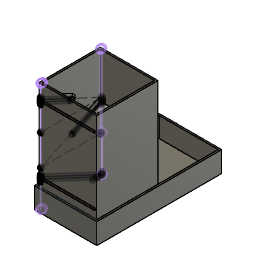
DiceTowerSlides (Autodesk Fusion 360 design; units mm, degrees)
Autodesk Fusion 360 part; units mm, degrees
sketch "Sketch1" plane through (0, 0, 0) normal (0, 1, 0) x (1, 0, 0)
  line L0 (30, 60) -> (-30, 60)
  line L1 (-30, 60) -> (-30, -60)
  line L2 (-30, -60) -> (30, -60)
  line L3 (30, -60) -> (30, 60)
  line L4 (30, 60) -> (-30, -60) construction
  line L5 (-30, 60) -> (30, -60) construction
  line L6 (28.33, 58.33) -> (-28.33, 58.33)
  line L7 (-28.33, 58.33) -> (-28.33, -58.33)
  line L8 (-28.33, -58.33) -> (28.33, -58.33)
  line L9 (28.33, -58.33) -> (28.33, 58.33)
  line L10 (28.33, 58.33) -> (-28.33, -58.33) construction
  line L11 (-28.33, 58.33) -> (28.33, -58.33) construction
  dimension "d3" = 120
  dimension "d4" = 60
  dimension "d5" = 1.67
  dimension "d6" = 1.67
  constraint horizontal L0
  constraint perpendicular L0 L1
  constraint parallel L0 L2
  constraint parallel L1 L3
  constraint coincident L4 origin
  constraint coincident L5 origin
  constraint horizontal L6
  constraint perpendicular L6 L7
  constraint parallel L6 L8
  constraint parallel L7 L9
  constraint coincident L10 origin
  constraint coincident L11 origin
  measures "d3" distance of L0.end L1.end
  measures "d4" distance of L1 L3
  measures "d5" distance of L1 L7
  measures "d6" distance of L0 L6
extrude "Extrude1" add sketch "Sketch1" along normal blind 20 makes body 1
extrude "Extrude2" add sketch "Sketch1" along normal blind 0.8 contours L6 L7 L8 L9 bodies 1
sketch "Sketch2" plane through (0, 0, 58.33) normal (0, 0, -1) x (-1, 0, 0)
  line L0 (-28.33, 0.8) -> (28.33, 0.8)
  line L1 (28.33, 0.8) -> (28.33, 20)
  line L2 (28.33, 20) -> (-28.33, 20)
  line L3 (-28.33, 20) -> (-28.33, 0.8)
sketch "Sketch2 (2)" plane through (0, 0.8, 0) normal (0, 1, 0) x (-1, 0, 0) in component "Tower"
  line L0 (-28.33, 58.33) -> (-28.33, -58.33)
  line L1 (-28.33, -58.33) -> (28.33, -58.33)
  line L2 (28.33, -58.33) -> (28.33, 58.33)
  line L3 (28.33, 58.33) -> (-28.33, 58.33)
  line L4 (28.33, 58.33) -> (-28.33, 58.33)
  line L5 (-28.33, 58.33) -> (28.33, 58.33) construction
  line L6 (28.33, 58.33) -> (28.33, -1.67) construction
  line L7 (28.33, -1.67) -> (-28.33, -1.67) construction
  line L8 (-28.33, -1.67) -> (-28.33, 58.33) construction
  line L9 (27.73, 57.73) -> (27.73, -1.07)
  line L10 (27.73, -1.07) -> (-27.73, -1.07)
  line L11 (-27.73, -1.07) -> (-27.73, 57.73)
  line L12 (-27.73, 57.73) -> (27.73, 57.73)
  line L13 (26.06, 0.6) -> (-26.06, 0.6)
  line L14 (-26.06, 0.6) -> (-26.06, 56.06)
  line L15 (-26.06, 56.06) -> (26.06, 56.06)
  line L16 (26.06, 56.06) -> (26.06, 0.6)
  point P0 (28.33, 58.33)
  point P1 (-28.33, 58.33)
  dimension "d39" = 60
  dimension "d43" = 0.6
  dimension "d44" = 1.67
  constraint horizontal L5
  constraint vertical L6
  constraint horizontal L7
  constraint vertical L8
  constraint coincident P0 L2.end
  constraint coincident P1 L0.start
  measures "d39" distance of P1 L7.end
extrude "Extrude2'" add sketch "Sketch2 (2)" along normal blind 105 separate body contours L9 L10 L11 L12 makes body 2 in component "Tower"
sketch "Sketch3" plane through (0, 0, -1.07) normal (0, 0, -1) x (-1, 0, 0) in component "Tower"
  line L0 (-27.73, 0.8) -> (27.73, 0.8)
  line L1 (27.73, 0.8) -> (27.73, 105.8)
  line L2 (27.73, 105.8) -> (-27.73, 105.8)
  line L3 (-27.73, 105.8) -> (-27.73, 0.8)
  line L4 (27.73, 0.8) -> (-27.73, 0.8)
  line L5 (-26.06, 0.8) -> (26.06, 0.8)
  line L6 (26.06, 0.8) -> (26.06, 35.8)
  line L7 (26.06, 35.8) -> (-26.06, 35.8)
  line L8 (-26.06, 35.8) -> (-26.06, 0.8)
  line L9 (26.06, 0.8) -> (26.06, 105.8)
  line L10 (-26.06, 0.8) -> (-26.06, 105.8)
  dimension "d49" = 35
  constraint horizontal L5
  constraint vertical L6
  constraint horizontal L7
  constraint vertical L8
  constraint coincident L0 L5.start
  constraint coincident L6 L5.end
  constraint coincident L5.start L10
  measures "d49" distance of L5 L7
extrude "Extrude3" cut sketch "Sketch3" against normal up to surface (1.67 mm away) contours L0 L4 L5 L6 L7 L8 L9 L10 bodies 2 in component "Tower"
sketch "Sketch6" plane through (-26.06, 0, 0) normal (1, 0, 0) x (0, 0, -1) in component "Tower"
  line L0 (-56.06, 0.8) -> (1.07, 0.8)
  line L1 (1.07, 0.8) -> (1.07, 35.8)
  line L2 (1.07, 35.8) -> (-0.6, 35.8)
  line L3 (-0.6, 35.8) -> (-0.6, 105.8)
  line L4 (-0.6, 105.8) -> (-56.06, 105.8)
  line L5 (1.07, 0.8) -> (-57.73, 28.2189)
  line L6 (-57.73, 26.0121) -> (-3.6624, 0.8)
  line L7 (-57.73, 30.0615) -> (1.07, 2.6426)
  line L8 (-57.73, 24.1695) -> (-7.614, 0.8)
  line L9 (-57.73, 0.8) -> (-57.73, 105.8)
  line L10 (-7.614, 0.8) -> (-3.6624, 0.8)
  line L11 (1.07, 2.6426) -> (1.07, 0.8)
  line L12 (-57.73, 30.0615) -> (-57.73, 28.2189)
  line L13 (-57.73, 26.0121) -> (-57.73, 24.1695)
  line L14 (-57.73, 27.9982) -> (0.5968, 0.8)
  line L15 (-57.73, 26.2328) -> (-3.1892, 0.8)
  line L16 (-57.73, 27.9982) -> (-57.73, 26.2328)
  line L17 (0.5968, 0.8) -> (-3.1892, 0.8)
  line L18 (1.07, 0.8) -> (1.07, 35.8)
  line L19 (-0.6, 35.8) -> (-0.6, 105.8)
  line L20 (-0.6, 35.8) -> (-57.73, 35.8) construction
  line L21 (1.07, 63.2189) -> (-57.73, 35.8) construction
  line L22 (1.07, 63.2189) -> (-27.73, 49.7892)
  line L23 (1.07, 62.9982) -> (-27.4642, 49.6925)
  line L24 (1.07, 61.2328) -> (-26.788, 48.2424)
  line L25 (1.07, 61.0121) -> (-26.8848, 47.9766)
  line L26 (1.07, 59.1695) -> (-26.179, 46.4631)
  line L27 (1.07, 65.0615) -> (-28.4358, 51.3028)
  line L28 (-26.179, 46.4631) -> (-26.8848, 47.9766)
  line L29 (-26.788, 48.2424) -> (-27.4642, 49.6925)
  line L30 (-28.4358, 51.3028) -> (-27.73, 49.7892)
  line L31 (-27.73, 49.7892) -> (-26.8848, 47.9766)
  line L32 (1.07, 0.8) -> (1.07, 105.8)
  line L33 (1.07, 62.9982) -> (1.07, 61.2328)
  line L34 (1.07, 63.2189) -> (1.07, 65.0615)
  line L35 (1.07, 61.0121) -> (1.07, 59.1695)
  arc A0 (-28.4358, 51.3028) -> (-26.179, 46.4631) centre (-27.3074, 48.8829) ccw
  line L36 (1.07, 65.0615) -> (-57.73, 65.0615) construction
  line L37 (1.07, 65.0615) -> (-57.73, 92.4804) construction
  line L38 (-57.73, 92.4804) -> (-28.93, 79.0508)
  line L39 (-57.73, 94.3231) -> (-28.2242, 80.5643)
  line L40 (-57.73, 92.2597) -> (-29.1958, 78.954)
  line L41 (-57.73, 90.4943) -> (-29.872, 77.5039)
  line L42 (-57.73, 90.2737) -> (-29.7752, 77.2381)
  line L43 (-57.73, 88.431) -> (-30.481, 75.7246)
  line L44 (-28.2242, 80.5643) -> (-28.93, 79.0508)
  line L45 (-29.1958, 78.954) -> (-29.872, 77.5039)
  line L46 (-29.7752, 77.2381) -> (-30.481, 75.7246)
  line L47 (-29.7752, 77.2381) -> (-28.93, 79.0508)
  arc A1 (-30.481, 75.7246) -> (-28.2242, 80.5643) centre (-29.3526, 78.1445) ccw
  dimension "d78" = 25
  dimension "d79" = 1.67
  dimension "d80" = 1.67
  dimension "d94" = 0.2
  dimension "d95" = 0.2
  dimension "d99" = 1.6
  dimension "d100" = 25
  dimension "d101" = 30
  dimension "d102" = 0.2
  dimension "d103" = 0.2
  dimension "d104" = 1.67
  dimension "d105" = 1.67
  dimension "d106" = 1.6
  dimension "d107" = 0.2
  dimension "d128" = 25
  dimension "d129" = 30
  dimension "d130" = 0.2
  dimension "d131" = 0.2
  dimension "d132" = 1.6
  dimension "d133" = 1.67
  dimension "d134" = 1.67
  dimension "d135" = 0.2
  constraint coincident L0.end L1.start
  constraint coincident L0 L6.end
  constraint parallel L5 L6
  constraint coincident L1 L7.end
  constraint coincident L0 L8.end
  constraint parallel L7 L8
  constraint parallel L5 L7
  constraint coincident L7.start L9
  constraint coincident L5.end L9
  constraint coincident L6.start L9
  constraint coincident L8.start L9
  constraint coincident L9 L14.start
  constraint coincident L0 L14.end
  constraint coincident L9 L15.start
  constraint coincident L0 L15.end
  constraint parallel L6 L15
  constraint parallel L6 L14
  constraint coincident L2.end L3.start
  constraint coincident L9 L20.end
  constraint perpendicular L9 L20
  constraint coincident L21 L22.end
  constraint parallel L24 L27
  constraint parallel L24 L25
  constraint parallel L25 L26
  constraint parallel L23 L26
  constraint parallel L22 L23
  constraint perpendicular L26 L28
  constraint coincident L25.end L28.end
  constraint perpendicular L24 L29
  constraint perpendicular L22 L30
  constraint collinear L28 L30
  constraint coincident L27.start L32
  constraint coincident L21.start L32
  constraint coincident L23.start L32
  constraint coincident L24.start L32
  constraint coincident L25.start L32
  constraint coincident L26.start L32
  constraint midpoint L31 A0.centre
  constraint coincident L9 L36.end
  constraint perpendicular L9 L36
  constraint coincident L9 L37.end
  constraint coincident L37 L38.end
  constraint coincident L9 L39.start
  constraint coincident L9 L40.start
  constraint coincident L9 L41.start
  constraint coincident L9 L42.start
  constraint coincident L9 L43.start
  constraint parallel L41 L42
  constraint parallel L41 L43
  constraint parallel L40 L43
  constraint parallel L39 L40
  constraint parallel L38 L39
  constraint perpendicular L43 L46
  constraint perpendicular L41 L45
  constraint perpendicular L39 L44
  constraint collinear L44 L46
  constraint midpoint L47 A1.centre
  measures "d78" angle of L0 L6
  measures "d79" distance of L6 L8
  measures "d80" distance of L5 L7
  measures "d94" distance of L5 L14
  measures "d95" distance of L6 L15
  measures "d99" distance of L14 L15
  measures "d100" angle of L20 L21
  measures "d101" distance of L9 L22.end
  measures "d102" distance of L22 L23
  measures "d103" distance of L24 L25
  measures "d104" distance of L25 L26
  measures "d105" distance of L21 L27
  measures "d106" distance of L23 L24
  measures "d107" distance of L29 L31
  measures "d128" angle of L36 L37
  measures "d129" distance of L32 L38.end
  measures "d130" distance of L38 L40
  measures "d131" distance of L41 L42
  measures "d132" distance of L40 L41
  measures "d133" distance of L42 L43
  measures "d134" distance of L38 L39
  measures "d135" distance of L45 L47
extrude "Extrude6" cut sketch "Sketch6" along normal up to surface (52.12 mm away) contours L0 L6 L9 L15 | L0 L9 L14 L15 L16 L17 | L0 L5 L9 L14 bodies 2 in component "Tower"
extrude "Extrude7" add sketch "Sketch6" along normal blind 1.67 contours L0 L6 L8 L9 L10 L13 | L1 L5 L7 L9 L11 L12 L18 L32 bodies 2 in component "Tower"
extrude "Extrude8" add sketch "Sketch6" against normal blind 1.67 from surface at 52.12 contours L0 L6 L8 L9 L10 L13 | L1 L5 L7 L9 L11 L12 L18 L32 bodies 2 in component "Tower"
extrude "Extrude9" add sketch "Sketch6" along normal up to surface (51.72 mm away) from surface at 0.2 separate body contours L0 L9 L14 L15 L16 L17 makes body 3 in component "Tower"
extrude "Extrude10" add sketch "Sketch6" along normal blind 1.67 contours L3 L19 L25 L26 L28 | L28 L30 L31 A0 | L3 L19 L22 L27 L30 bodies 2 in component "Tower"
fillet "Fillet4" radius 2 1 edges at (-26.06, 15.9627, 27.495) on bodies 2 in component "Tower"
extrude "Extrude11" cut sketch "Sketch6" along normal up to surface (52.12 mm away) contours L3 L19 L24 L25 L32 | L3 L19 L23 L24 L32 L33 | L3 L19 L22 L23 L32 bodies 2 in component "Tower"
fillet "Fillet5" radius 2 3 edges at (-26.06, 52.4269, 13.3895) (-26.06, 47.7545, 29.7272) (-26.06, 57.7928, 14.5179) on bodies 2 in component "Tower"
extrude "Extrude12" add sketch "Sketch6" against normal blind 1.67 from surface at 52.12 contours L3 L19 L25 L26 L28 | L28 L30 L31 A0 | L3 L19 L22 L27 L30 bodies 2 in component "Tower"
fillet "Fillet6" radius 2 3 edges at (26.06, 57.7928, 14.5179) (26.06, 47.7545, 29.7272) (26.06, 52.4269, 13.3895) on bodies 2 in component "Tower"
extrude "Extrude13" add sketch "Sketch6" along normal up to surface (51.72 mm away) from surface at 0.2 separate body contours L3 L19 L23 L24 L32 L33 | L3 L19 L23 L24 L29 makes body 4 in component "Tower"
extrude "Extrude14" cut sketch "Sketch6" along normal up to surface (52.12 mm away) contours L9 L38 L40 L41 L42 L45 L47 | L9 L40 L41 L45 bodies 2 in component "Tower"
extrude "Extrude15" add sketch "Sketch6" along normal blind 1.67 contours L9 L42 L43 L46 | L44 L46 L47 A1 | L9 L38 L39 L44 bodies 2 in component "Tower"
extrude "Extrude16" add sketch "Sketch6" against normal blind 1.67 from surface at 52.12 contours L9 L42 L43 L46 | L44 L46 L47 A1 | L9 L38 L39 L44 bodies 2 in component "Tower"
fillet "Fillet7" radius 2 3 edges at (26.06, 81.6885, 43.2705) (26.06, 77.0161, 26.9328) (26.06, 87.0543, 42.1421) on bodies 2 in component "Tower"
fillet "Fillet8" radius 2 3 edges at (-26.06, 87.0543, 42.1421) (-26.06, 77.0161, 26.9328) (-26.06, 81.6885, 43.2705) on bodies 2 in component "Tower"
extrude "Extrude17" add sketch "Sketch6" along normal up to surface (51.72 mm away) from surface at 0.2 separate body contours L9 L40 L41 L45 makes body 5 in component "Tower"
fillet "Fillet9" radius 2 1 edges at (26.06, 15.9627, 27.495) on bodies 2 in component "Tower"
component "Tower" placed x (1, 0, 0) y (0, 1, 0) z (0, 0, 1) at (0, 0, 0)
equation "d44 = ( 1.67 ) * 1 mm"
equation "d45 = 140.00 mm - 35 mm"
